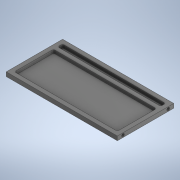
# Autodesk Inventor part: Cockpit_front_frame
Saved by Autodesk Inventor 2020 (Build 240168000, 168)
## iProperties
Part Number: Cockpit_front_frame
Material: アセタール樹脂、黒
Document SubType Name: Modeling
Designer: Masato Kubotera
Density: 1.425 g/cm^3
Appearance: 滑らか - 黒
Description: POM T5
Mass: 23.89 g
Surface Area: 240.544 cm^2
Volume: 16.7649 cm^3
Author: Masato Kubotera
Autodesk Inventor part; units mm, degrees
ref_plane "XZ Plane" through (0, 0, 0) normal (0, 1, 0) x (-1, 0, 0)
ref_plane "XY Plane" through (0, 0, 0) normal (0, 0, 1) x (1, 0, 0)
derived "Cockpit_side_frame.ipt"
sketch "スケッチ2" plane through (0, 0, 0) normal (0, 1, 0) x (-1, 0, 0)
  line L0 (-23.5, -22.5) -> (-28.5, -27.5)
  line L1 (-28.5, -27.5) -> (-28.5, -91)
  line L2 (-28.5, -91) -> (-23.5, -96)
  line L3 (-23.5, -96) -> (35.75, -96)
  line L4 (37.75, -98) -> (37.75, -131)
  line L5 (37.75, -131) -> (42.75, -136)
  line L6 (42.75, -136) -> (83.5, -136)
  line L7 (88.5, -131) -> (88.5, -20)
  line L8 (88.5, -20) -> (86, -17.5)
  line L9 (86, -17.5) -> (80.25, -17.5)
  line L10 (80.25, -17.5) -> (80.25, -21.0151)
  line L11 (78.7651, -22.5) -> (73.9849, -22.5)
  line L12 (72.5, -21.0151) -> (72.5, -17.5)
  line L13 (72.5, -17.5) -> (64.5, -17.5)
  line L14 (64.5, -17.5) -> (64.5, -21.0151)
  line L15 (63.0151, -22.5) -> (-23.5, -22.5)
  line L16 (-25.25, -25) -> (-20.25, -25) construction
  line L17 (-20.25, -25) -> (-20.25, -93.5) construction
  line L18 (-20.25, -93.5) -> (-25.25, -93.5) construction
  line L19 (-25.25, -93.5) -> (-25.25, -25) construction
  line L20 (-26, -25) -> (-25.25, -25) construction
  line L21 (-25.25, -93.5) -> (-26, -93.5) construction
  line L22 (-26, -93.5) -> (-26, -25) construction
  line L23 (-20.25, -93.5) -> (80.25, -93.5) construction
  line L24 (-20.25, -88.5) -> (80.25, -88.5) construction
  line L25 (80.25, -22.5) -> (80.25, -90.5) construction
  line L26 (80.25, -90.5) -> (85.25, -90.5) construction
  line L27 (85.25, -90.5) -> (85.25, -22.5) construction
  line L28 (80.25, -88.5) -> (80.25, -93.5) construction
  line L29 (80.25, -91) -> (85.25, -91) construction
  line L30 (85.25, -91) -> (85.25, -133.5) construction
  line L31 (80.25, -91) -> (80.25, -133.5) construction
  line L32 (80.25, -133.5) -> (85.25, -133.5) construction
  line L33 (40.25, -133.5) -> (40.25, -128.5) construction
  line L34 (40.25, -128.5) -> (40.25, -93.5) construction
  line L35 (45.25, -93.5) -> (45.25, -128.5) construction
  line L36 (40.25, -128.5) -> (45.25, -128.5) construction
  line L37 (42.75, -128.5) -> (42.75, -93.5) construction
  line L38 (40.25, -128.5) -> (79.1145, -128.5) construction
  line L39 (79.1145, -128.5) -> (79.1145, -133.5) construction
  line L40 (79.1145, -133.5) -> (40.25, -133.5) construction
  line L41 (40.25, -131) -> (79.1145, -131) construction
  line L42 (82.75, -91) -> (82.75, -133.5) construction
  circle A0 centre (82.75, -131) radius 2
  arc A1 (80.25, -128.5) -> (85.25, -128.5) centre (82.75, -131) ccw construction
  line L43 (80.25, -91) -> (-20.25, -91) construction
  line L44 (42.75, -111) -> (45.25, -111) construction
  line L45 (59.6822, -128.5) -> (59.6822, -131) construction
  line L46 (42.7, -115.5651) -> (42.7, -106.4349)
  line L47 (45.3, -107.05) -> (45.3, -114.95)
  line L48 (45.3, -117.05) -> (42.7, -104.95) construction
  line L49 (42.7, -117.05) -> (45.3, -104.95) construction
  line L50 (55.7322, -128.45) -> (63.6322, -128.45)
  line L51 (64.2473, -131.05) -> (55.1172, -131.05)
  line L52 (53.6322, -128.45) -> (65.7322, -131.05) construction
  line L53 (65.7322, -128.45) -> (53.6322, -131.05) construction
  line L54 (42.75, -105) -> (45.25, -105) construction
  line L55 (42.75, -117) -> (45.25, -117) construction
  arc A2 (44.1849, -104.95) -> (42.7, -106.4349) centre (43.4425, -105.6925) ccw
  arc A3 (45.3, -107.05) -> (45.3, -104.95) centre (45.3, -106) ccw
  arc A4 (42.7, -115.5651) -> (44.1849, -117.05) centre (43.4425, -116.3075) ccw
  arc A5 (45.3, -117.05) -> (45.3, -114.95) centre (45.3, -116) ccw
  line L56 (53.6822, -131) -> (53.6822, -128.5) construction
  line L57 (65.6822, -128.5) -> (65.6822, -131) construction
  arc A6 (53.6322, -129.5651) -> (55.1172, -131.05) centre (54.3747, -130.3075) ccw
  arc A7 (55.7322, -128.45) -> (53.6322, -128.45) centre (54.6822, -128.45) ccw
  arc A8 (64.2473, -131.05) -> (65.7322, -129.5651) centre (64.9898, -130.3075) ccw
  arc A9 (65.7322, -128.45) -> (63.6322, -128.45) centre (64.6822, -128.45) ccw
  line L58 (53.6322, -129.5651) -> (53.6322, -128.45)
  line L59 (65.7322, -128.45) -> (65.7322, -129.5651)
  line L60 (44.1849, -104.95) -> (45.3, -104.95)
  line L61 (45.3, -117.05) -> (44.1849, -117.05)
  circle A10 centre (47.6822, -131) radius 1.6
  line L62 (85.25, -22.5) -> (85.25, -17.5) construction
  line L63 (86, -17.5) -> (86, -90.5) construction
  line L64 (86, -90.5) -> (85.25, -90.5) construction
  line L65 (-13.5, -82.5) -> (-13.5, -61)
  arc A11 (-13.5, -82.5) -> (-11.5, -84.5) centre (-11.5, -82.5) ccw
  line L66 (45.5, -84.5) -> (-11.5, -84.5)
  arc A12 (45.5, -84.5) -> (47.5, -82.5) centre (45.5, -82.5) ccw
  line L67 (47.5, -61) -> (47.5, -82.5)
  arc A13 (47.5, -61) -> (45.5, -59) centre (45.5, -61) ccw
  line L68 (-11.5, -59) -> (45.5, -59)
  arc A14 (-11.5, -59) -> (-13.5, -61) centre (-11.5, -61) ccw
  line L69 (30, -88.5) -> (30, -91) construction
  line L70 (82.75, -22.5) -> (82.75, -90.5) construction
  circle A15 centre (82.75, -34) radius 1.6
  circle A16 centre (82.75, -34) radius 3
  circle A17 centre (82.75, -79) radius 3
  circle A18 centre (82.75, -79) radius 1.6
  line L71 (85.25, -22.5) -> (80.25, -22.5) construction
  arc A19 (85.25, -91) -> (80.25, -91) centre (82.75, -131) ccw construction
  circle A20 centre (47.6822, -131) radius 3
  circle A21 centre (42.75, -99) radius 1.6
  circle A22 centre (42.75, -99) radius 3
  line L72 (5, -88.5) -> (5, -91) construction
  line L73 (55, -88.5) -> (55, -91) construction
  line L74 (53.5651, -91.05) -> (6.4349, -91.05)
  line L75 (4.95, -89.5651) -> (4.95, -88.45)
  line L76 (7.05, -88.45) -> (52.95, -88.45)
  line L77 (55.05, -88.45) -> (55.05, -89.5651)
  line L78 (55.05, -91.05) -> (4.95, -88.45) construction
  line L79 (4.95, -91.05) -> (55.05, -88.45) construction
  arc A23 (7.05, -88.45) -> (4.95, -88.45) centre (6, -88.45) ccw
  arc A24 (4.95, -89.5651) -> (6.4349, -91.05) centre (5.6925, -90.3075) ccw
  arc A25 (53.5651, -91.05) -> (55.05, -89.5651) centre (54.3075, -90.3075) ccw
  arc A26 (55.05, -88.45) -> (52.95, -88.45) centre (54, -88.45) ccw
  line L80 (-20.25, -41) -> (80.25, -41) construction
  line L81 (80.25, -36) -> (-20.25, -36) construction
  line L82 (-20.25, -36) -> (-20.25, -41) construction
  line L83 (-20.25, -38.5) -> (80.25, -38.5) construction
  line L84 (30, -41) -> (30, -36) construction
  line L85 (53.5651, -35.95) -> (6.4349, -35.95)
  line L86 (6.4349, -41.05) -> (53.5651, -41.05)
  line L87 (55.05, -35.95) -> (4.95, -41.05) construction
  line L88 (4.95, -35.95) -> (55.5723, -41.1032) construction
  arc A27 (6.4349, -35.95) -> (4.95, -37.4349) centre (5.6925, -36.6925) ccw
  arc A28 (4.95, -39.5651) -> (6.4349, -41.05) centre (5.6925, -40.3075) ccw
  arc A29 (55.05, -37.4349) -> (53.5651, -35.95) centre (54.3075, -36.6925) ccw
  arc A30 (53.5651, -41.05) -> (55.05, -39.5651) centre (54.3075, -40.3075) ccw
  line L89 (5, -41) -> (5, -36) construction
  line L90 (55, -36) -> (55, -41) construction
  line L91 (4.95, -37.4349) -> (4.95, -39.5651)
  line L92 (55.05, -39.5651) -> (55.05, -37.4349)
  circle A31 centre (-2.5, -38.5) radius 1.6
  circle A32 centre (-2.5, -38.5) radius 3
  circle A33 centre (62.5, -38.5) radius 1.6
  circle A34 centre (62.5, -38.5) radius 3
  line L93 (-25.25, -49.25) -> (-26, -49.25) construction
  line L94 (-25.25, -69.25) -> (-26, -69.25) construction
  line L95 (-26, -59.25) -> (-25.25, -59.25) construction
  line L96 (-22.75, -25) -> (-22.75, -93.5) construction
  arc A35 (63.0151, -22.5) -> (64.5, -21.0151) centre (63.7575, -21.7575) ccw
  arc A36 (72.5, -21.0151) -> (73.9849, -22.5) centre (73.2425, -21.7575) ccw
  line L97 (56.75, -22.5) -> (56.75, -32.5) construction
  line L98 (56.75, -32.5) -> (80.25, -32.5) construction
  line L99 (80.25, -32.5) -> (80.25, -22.5) construction
  line L100 (68.5, -17.5) -> (68.5, -32.5) construction
  line L101 (60.5, -22.5) -> (60.5, -17.5) construction
  line L102 (76.5, -22.5) -> (76.5, -17.5) construction
  circle A37 centre (-22.75, -31.75) radius 1.6
  circle A38 centre (-22.75, -31.75) radius 3
  circle A39 centre (-22.75, -86.75) radius 1.6
  circle A40 centre (-22.75, -86.75) radius 3
  line L103 (64.5, -22.5) -> (72.5, -22.5)
  line L104 (85.25, -17.5) -> (52.5, -17.5) construction
  line L105 (52.5, -17.5) -> (52.5, -22.5) construction
  circle A41 centre (82.75, -98.5) radius 1.475
  circle A42 centre (82.75, -103.5) radius 1.475
  circle A43 centre (82.75, -108.5) radius 1.475
  line L106 (49.75, -93.5) -> (75.75, -93.5)
  line L107 (77.75, -95.5) -> (77.75, -124)
  line L108 (75.75, -126) -> (49.75, -126)
  line L109 (47.75, -124) -> (47.75, -95.5)
  arc A44 (49.75, -93.5) -> (47.75, -95.5) centre (49.75, -95.5) ccw
  arc A45 (47.75, -124) -> (49.75, -126) centre (49.75, -124) ccw
  arc A46 (75.75, -126) -> (77.75, -124) centre (75.75, -124) ccw
  arc A47 (77.75, -95.5) -> (75.75, -93.5) centre (75.75, -95.5) ccw
  arc A48 (37.75, -98) -> (35.75, -96) centre (35.75, -98) ccw
  circle A49 centre (-13.5, -55) radius 1.75
  circle A50 centre (-13.5, -55) radius 2
  line L110 (74.85, -78.65) -> (65.65, -78.65) construction
  line L111 (65.65, -78.65) -> (65.65, -64.85) construction
  line L112 (65.65, -64.85) -> (74.85, -64.85) construction
  line L113 (74.85, -64.85) -> (74.85, -78.65) construction
  line L114 (74.85, -78.65) -> (65.65, -64.85) construction
  line L115 (65.65, -78.65) -> (74.85, -64.85) construction
  line L116 (64.95, -64.2) -> (75.55, -64.2) construction
  line L117 (75.55, -64.2) -> (75.55, -79.3) construction
  line L118 (75.55, -79.3) -> (64.95, -79.3) construction
  line L119 (64.95, -79.3) -> (64.95, -64.2) construction
  line L120 (64.95, -64.2) -> (75.55, -79.3) construction
  line L121 (75.55, -64.2) -> (64.95, -79.3) construction
  line L122 (66.3849, -64.15) -> (74.1151, -64.15)
  line L123 (75.6, -65.6349) -> (75.6, -77.8651)
  line L124 (75.6, -79.35) -> (64.9, -64.15) construction
  line L125 (64.9, -79.35) -> (75.6, -64.15) construction
  line L126 (74.9, -78.7) -> (65.6, -64.8) construction
  line L127 (65.6, -78.7) -> (74.9, -64.8) construction
  arc A51 (66.3849, -64.15) -> (64.9, -65.6349) centre (65.6425, -64.8925) ccw
  arc A52 (67.0849, -64.8) -> (65.6, -66.2849) centre (66.3425, -65.5425) ccw
  line L128 (64.9, -71.75) -> (75.6, -71.75) construction
  line L129 (70.25, -64.15) -> (70.25, -78.7063) construction
  arc A53 (75.6, -65.6349) -> (74.1151, -64.15) centre (74.8575, -64.8925) ccw
  arc A54 (74.9, -66.2849) -> (73.4151, -64.8) centre (74.1575, -65.5425) ccw
  arc A55 (65.6, -77.2151) -> (67.0849, -78.7) centre (66.3425, -77.9575) ccw
  arc A56 (64.9, -77.8651) -> (66.3849, -79.35) centre (65.6425, -78.6075) ccw
  arc A57 (73.4151, -78.7) -> (74.9, -77.2151) centre (74.1575, -77.9575) ccw
  arc A58 (74.1151, -79.35) -> (75.6, -77.8651) centre (74.8575, -78.6075) ccw
  line L130 (67.0849, -64.8) -> (73.4151, -64.8)
  line L131 (74.9, -66.2849) -> (74.9, -77.2151)
  line L132 (64.9, -77.8651) -> (64.9, -65.6349)
  line L133 (65.6, -77.2151) -> (65.6, -66.2849)
  line L134 (73.4151, -78.7) -> (67.0849, -78.7)
  line L135 (74.1151, -79.35) -> (66.3849, -79.35)
  line L136 (-13.5, -71.75) -> (47.5, -71.75) construction
  line L137 (82.75, -56.5) -> (85.25, -56.5) construction
  line L138 (86, -54) -> (85.25, -54) construction
  line L139 (82.7, -69.45) -> (82.7, -43.55)
  line L140 (85.3057, -71.616) -> (82.7, -41.45) construction
  line L141 (82.7, -71.55) -> (85.3, -41.45) construction
  arc A59 (82.7, -41.45) -> (82.7, -43.55) centre (82.7, -42.5) ccw
  arc A60 (85.3, -42.9349) -> (83.8151, -41.45) centre (84.5575, -42.1925) ccw
  arc A61 (82.7, -69.45) -> (82.7, -71.55) centre (82.7, -70.5) ccw
  arc A62 (83.8151, -71.55) -> (85.3, -70.0651) centre (84.5575, -70.8075) ccw
  line L142 (82.75, -41.5) -> (85.25, -41.5) construction
  line L143 (82.75, -71.5) -> (85.25, -71.5) construction
  arc A63 (86.25, -47.1801) -> (85.3, -46.1348) centre (85.2, -47.1801) ccw
  line L144 (86.25, -47.1801) -> (86.25, -65.8199)
  line L145 (85.25, -46.5) -> (86, -46.5) construction
  line L146 (85.25, -66.5) -> (86, -66.5) construction
  arc A64 (85.3, -66.8652) -> (86.25, -65.8199) centre (85.2, -65.8199) ccw
  line L147 (85.3, -42.9349) -> (85.3, -46.1348)
  line L148 (85.3, -66.8652) -> (85.3, -70.0651)
  line L149 (83.8151, -71.55) -> (82.7, -71.55)
  line L150 (82.7, -41.45) -> (83.8151, -41.45)
  line L151 (83.5, -136) -> (88.5, -131)
  arc A65 (78.7651, -22.5) -> (80.25, -21.0151) centre (79.5075, -21.7575) ccw
  circle A66 centre (82.75, -93.5) radius 2
  circle A67 centre (82.75, -93.5) radius 4 construction
  arc A68 (-24.15, -49.25) -> (-26.25, -49.25) centre (-25.2, -49.25) ccw
  line L152 (-26, -49.25) -> (-26.25, -49.25) construction
  line L153 (-26.25, -49.25) -> (-26.25, -69.25)
  line L154 (-24.15, -49.25) -> (-24.15, -69.25)
  arc A69 (-26.25, -69.25) -> (-24.15, -69.25) centre (-25.2, -69.25) ccw
  point P0 (0, 0)
  point P1 (-25.7227, -96)
  point P2 (-23.5, -22.5)
  point P3 (44, -111)
  point P4 (59.6822, -129.75)
  point P5 (30, -89.75)
  point P6 (30, -38.5)
  point P7 (4.95, -41.05)
  point P8 (52.5, -22)
  point P9 (70.25, -71.75)
  point P10 (70.25, -71.75)
  point P11 (84, -56.5)
  point P12 (80.25, -22.5)
  dimension "d1" = 25.25
  dimension "d2" = 5
  measures "d1" distance from line of L19 point (0, 0)
  measures "d2" distance of L16.start L16.end
ref_plane "作業平面1" through (25.25, 0, 0) normal (1, 0, 0) x (0, 1, 0)
sketch "スケッチ3" plane through (25.25, 0, 0) normal (1, 0, 0) x (0, 1, 0)
  line L0 (-135, -25) -> (0, -25)
  line L1 (0, -93.5) -> (-135, -93.5)
  line L2 (0, -25) -> (0, -93.5)
  line L3 (0, -75.7349) -> (0, -93.5)
  line L4 (-67.5, -25) -> (-67.5, -93.5) construction
  line L5 (-135, -25) -> (-135, -93.5)
  line L6 (-7, -30) -> (-128, -30)
  line L7 (-130, -32) -> (-130, -34)
  line L8 (-128, -36) -> (-7, -36)
  line L9 (-5, -34) -> (-5, -32)
  line L10 (-5, -30) -> (-130, -36) construction
  line L11 (-130, -30) -> (-5, -36) construction
  line L12 (-7, -88.5) -> (-128, -88.5)
  line L13 (-130, -86.5) -> (-130, -43)
  line L14 (-128, -41) -> (-7, -41)
  line L15 (-5, -43) -> (-5, -86.5)
  line L16 (-5, -88.5) -> (-130, -41) construction
  line L17 (-130, -88.5) -> (-5, -41) construction
  arc A0 (-128, -30) -> (-130, -32) centre (-128, -32) ccw
  arc A1 (-130, -34) -> (-128, -36) centre (-128, -34) ccw
  arc A2 (-7, -36) -> (-5, -34) centre (-7, -34) ccw
  arc A3 (-5, -32) -> (-7, -30) centre (-7, -32) ccw
  arc A4 (-5, -43) -> (-7, -41) centre (-7, -43) ccw
  arc A5 (-128, -41) -> (-130, -43) centre (-128, -43) ccw
  arc A6 (-130, -86.5) -> (-128, -88.5) centre (-128, -86.5) ccw
  arc A7 (-7, -88.5) -> (-5, -86.5) centre (-7, -86.5) ccw
  point P0 (0, 0)
  point P1 (-135, -25)
  point P2 (-135, -93.5)
  point P3 (-67.5, -33)
  point P4 (-67.5, -64.75)
  point P5 (0, -36)
  point P6 (0, -36)
  point P7 (0, -36)
  point P8 (0, -41)
  point P9 (0, -41)
  point P10 (0, -41)
  dimension "d6" = 135
  dimension "d19" = 2
  dimension "d20" = 5
  dimension "d21" = 5
  dimension "d22" = 5
  constraints: 36 end point, 21 point on line, 16 point on circle, 16 tangent, 8 centre point, 7 equal radius, 6 midpoint, 5 parallel, 4 coincident, 4 perpendicular, 3 horizontal, 3 symmetric about line
  measures "d6" distance of L0.start L0.end
  measures "d19" radius of A0
  measures "d20" distance between parallel lines of L2 L9
  measures "d21" distance between parallel lines of L6 L0
  measures "d22" distance between parallel lines of L1 L12
extrude "押し出し1" add sketch "スケッチ3" against normal blind 5
hole "穴1" at (22.75, 0, -31.75) at (22.75, 0, -86.75) direction (0, -1, 0) diameter 3.4587 depth 4 thread size "M4x0.5" class "6H" standard "ANSI Metric M Profile"
ref_plane "作業平面2" through (25.25, -67.5, -25) normal (0, 1, 0) x (-1, 0, 0)
mirror "ミラー1" about plane through (25.25, -67.5, -25) normal (0, 1, 0) of "穴1"
extrude "押し出し3" add sketch "スケッチ3" against normal blind 1 contours A3 L9 A2 L8 A1 L7 A0 L6 | L12 A6 L13 A5 L14 A4 L15 A7
equation "\"d8\" = d2"
equation "\"d4\" = d1"
